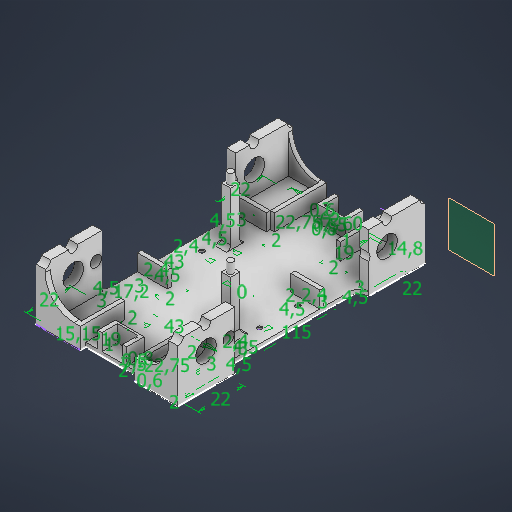
# Autodesk Inventor part: MainBody_thin
Saved by Autodesk Inventor 2026.1 (Build 301233000, 233)
## iProperties
Created: 2026-05-04
Part Number: MainBody_thin
Material: Generic
Document SubType Name: Modeling
Designer: 25adoh
Density: 1 g/cm^3
Appearance: Default
Author: 25adoh
Autodesk Inventor part; units mm, degrees
ref_plane "YZ Plane" through (0, 0, 0) normal (1, 0, 0) x (0, 1, 0)
ref_plane "XZ Plane" through (0, 0, 0) normal (0, 1, 0) x (-1, 0, 0)
ref_plane "XY Plane" through (0, 0, 0) normal (0, 0, 1) x (1, 0, 0)
sketch "Sketch1" plane through (0, 0, 0) normal (0, 1, 0) x (-1, 0, 0)
  line L0 (0, 0) -> (-60, 0)
  line L1 (-60, 0) -> (-60, -115)
  line L2 (-60, -115) -> (0, -115)
  line L3 (0, -115) -> (0, 0)
  line L4 (0, 0) -> (4.5, 0)
  line L5 (4.5, 0) -> (4.5, -22)
  line L6 (4.5, -22) -> (0, -22)
  line L7 (0, -22) -> (0, 0)
  line L8 (-60, 0) -> (-64.5, 0)
  line L9 (-64.5, 0) -> (-64.5, -22)
  line L10 (-64.5, -22) -> (-60, -22)
  line L11 (-60, -22) -> (-60, 0)
  line L12 (0, -115) -> (4.5, -115)
  line L13 (4.5, -115) -> (4.5, -93)
  line L14 (4.5, -93) -> (0, -93)
  line L15 (0, -93) -> (0, -115)
  line L16 (-60, -115) -> (-64.5, -115)
  line L17 (-64.5, -115) -> (-64.5, -93)
  line L18 (-64.5, -93) -> (-60, -93)
  line L19 (-60, -93) -> (-60, -115)
  line L20 (-44.8503, -96.0032) -> (-42.8503, -96.0032)
  line L21 (-42.8503, -96.0032) -> (-42.8503, -115)
  line L22 (-15.15, 0) -> (-15.15, -19)
  line L23 (-15.15, -19) -> (-17.15, -19)
  line L24 (-17.15, -19) -> (-17.15, 0)
  line L25 (-17.15, 0) -> (-15.15, 0)
  line L26 (-16.5, -115) -> (-14.5, -115)
  line L27 (-45.2, -115) -> (-42.8503, -115)
  line L28 (-46, -72.8) -> (-60, -72.8)
  line L29 (-46, -72.8) -> (-46, -70.8)
  line L30 (-46, -70.8) -> (-60, -70.8)
  line L31 (0, 0) -> (-15.15, 0)
  line L32 (-14.5, -42.2) -> (0, -42.2)
  line L33 (-43.5, 0) -> (-43.5, -22.75)
  line L34 (-45.5, 0) -> (-45.5, -22.75)
  line L35 (-45.5, -22.75) -> (-43.5, -22.75)
  line L36 (-43.5, -22.75) -> (-43.5, -24.75)
  line L37 (-43.5, 0) -> (-45.5, 0)
  line L38 (-43.5, -24.75) -> (-60, -24.75)
  line L39 (-45.5, -22.75) -> (-60, -22.75)
  line L40 (-14.5, -115) -> (-14.5, -92.25)
  line L41 (-14.5, -92.25) -> (0, -92.25)
  line L42 (-16.5, -115) -> (-16.5, -92.25)
  line L43 (-16.5, -92.25) -> (-14.5, -92.25)
  line L44 (-16.5, -92.25) -> (-16.5, -90.25)
  line L45 (-16.5, -90.25) -> (0, -90.25)
  line L46 (-45.5, 0) -> (-45.5, 0.6)
  line L47 (-60, 0) -> (-60, 0.6)
  line L48 (-60, 0.6) -> (-45.5, 0.6)
  line L49 (-60, 0.6) -> (-60, 2.6)
  line L50 (-60, 2.6) -> (-43.5, 2.6)
  line L51 (-43.5, 2.6) -> (-43.5, 0)
  line L52 (-16.5, -115) -> (-16.5, -115.6)
  line L53 (-16.5, -115.6) -> (0, -115.6)
  line L54 (-16.5, -115.6) -> (-16.5, -117.6)
  line L55 (-16.5, -117.6) -> (0, -117.6)
  line L56 (0, -117.6) -> (0, -115.6)
  line L57 (0, -115.6) -> (0, -115)
  line L58 (-14.5, -115) -> (-14.5, -115.6)
  line L59 (-17.15, 0) -> (0, 0)
  line L60 (0, 0) -> (0, 2.6)
  line L61 (0, 2.6) -> (-17.15, 2.6)
  line L62 (-17.15, 2.6) -> (-17.15, 0)
  line L63 (-42.8503, -115) -> (-60, -115)
  line L64 (-60, -115) -> (-60, -117.6)
  line L65 (-60, -117.6) -> (-42.8503, -117.6)
  line L66 (-42.8503, -117.6) -> (-42.8503, -115)
  line L67 (-44.8503, -96.0032) -> (-44.8503, -115)
  line L68 (-14.5, -42.2) -> (-14.5, -44.2)
  line L69 (-14.5, -44.2) -> (0, -44.2)
  line L70 (-35, -115) -> (-35, 0)
  line L71 (-64.5, -22) -> (-60, -22)
  line L72 (-60, -22) -> (-60, -25)
  line L73 (-60, -25) -> (-64.5, -25)
  line L74 (-64.5, -25) -> (-64.5, -22)
  line L75 (-64.5, -93) -> (-60, -93)
  line L76 (-60, -93) -> (-60, -90)
  line L77 (-60, -90) -> (-64.5, -90)
  line L78 (-64.5, -90) -> (-64.5, -93)
  line L79 (4.5, -22) -> (0, -22)
  line L80 (0, -22) -> (0, -25)
  line L81 (0, -25) -> (4.5, -25)
  line L82 (4.5, -25) -> (4.5, -22)
  line L83 (4.5, -93) -> (0, -93)
  line L84 (0, -93) -> (0, -90)
  line L85 (0, -90) -> (4.5, -90)
  line L86 (4.5, -90) -> (4.5, -93)
  line L87 (-64.5, 0) -> (-60, 0)
  line L88 (-60, 0) -> (-60, 2.6)
  line L89 (-60, 2.6) -> (-64.5, 2.6)
  line L90 (-64.5, 2.6) -> (-64.5, 0)
  line L91 (0, 2.6) -> (4.5, 2.6)
  line L92 (4.5, 2.6) -> (4.5, 0)
  line L93 (4.5, 0) -> (0, 0)
  line L94 (0, 0) -> (0, 2.6)
  line L95 (0, -117.6) -> (4.5, -117.6)
  line L96 (4.5, -117.6) -> (4.5, -115)
  line L97 (4.5, -115) -> (0, -115)
  line L98 (0, -115) -> (0, -117.6)
  line L99 (-64.5, -115) -> (-60, -115)
  line L100 (-60, -115) -> (-60, -117.6)
  line L101 (-60, -117.6) -> (-64.5, -117.6)
  line L102 (-64.5, -117.6) -> (-64.5, -115)
  line L103 (-25, 0) -> (-35, 0)
  line L104 (-35, 0) -> (-35, -7.5)
  line L105 (-35, -7.5) -> (-25, -7.5)
  line L106 (-25, -7.5) -> (-25, 0)
  line L107 (-35, -7.5) -> (-35, -6.7)
  line L108 (-35, -5.7) -> (-35, -6.7)
  line L109 (-25, 0) -> (-23, 0)
  line L110 (-35, -7.5) -> (-37, -7.5)
  line L111 (-37, -7.5) -> (-37, 0)
  line L112 (-37, 0) -> (-35, 0)
  line L113 (-35, 0) -> (-35, -7.5)
  line L114 (-35, -6.7) -> (-35.3, -6.7)
  line L115 (-35, -6.5) -> (-35, -6.7)
  line L116 (-37, -7.5) -> (-23, -7.5)
  line L117 (-23, -8.5) -> (-37, -8.5)
  line L118 (-37, -8.5) -> (-37, -7.5)
  line L119 (-35, -6.7) -> (-35.5, -6.7)
  line L120 (-35.5, -6.7) -> (-35.5, -5.7)
  line L121 (-35.5, -5.7) -> (-35, -5.7)
  line L122 (-35, -5.7) -> (-35, -6.7)
  line L123 (-15.15, 0) -> (0, 0)
  line L124 (0, -25) -> (0, -42.2)
  line L125 (-23, -8.5) -> (-23, 0)
  line L126 (-25, -115) -> (-25, 0)
  circle A0 centre (-7, -66.5) radius 1.2
  circle A1 centre (-7, -48.5) radius 1.2
  circle A2 centre (-53.3, -48.2) radius 1.2
  circle A3 centre (-53.3, -66.8) radius 1.2
  line L127 (-51.5, -79) -> (-8.5, -79)
  line L128 (-8.5, -79) -> (-8.5, -36)
  line L129 (-8.5, -36) -> (-51.5, -36)
  line L130 (-51.5, -36) -> (-51.5, -79)
  line L131 (-51.5, -79) -> (-8.5, -36) construction
  line L132 (-8.5, -79) -> (-51.5, -36) construction
  circle A4 centre (-11.25, -38.75) radius 1.5
  circle A5 centre (-11.25, -38.75) radius 2.25
  line L133 (-9, -41) -> (-13.5, -41)
  line L134 (-13.5, -41) -> (-13.5, -36.5)
  line L135 (-13.5, -36.5) -> (-9, -36.5)
  line L136 (-9, -36.5) -> (-9, -41)
  circle A6 centre (-48.75, -38.75) radius 1.5
  circle A7 centre (-48.75, -38.75) radius 2.25
  line L137 (-51, -41) -> (-46.5, -41)
  line L138 (-46.5, -41) -> (-46.5, -36.5)
  line L139 (-46.5, -36.5) -> (-51, -36.5)
  line L140 (-51, -36.5) -> (-51, -41)
  circle A8 centre (-48.75, -76.25) radius 1.5
  circle A9 centre (-48.75, -76.25) radius 2.25
  line L141 (-46.5, -74) -> (-51, -74)
  line L142 (-51, -74) -> (-51, -78.5)
  line L143 (-51, -78.5) -> (-46.5, -78.5)
  line L144 (-46.5, -78.5) -> (-46.5, -74)
  circle A10 centre (-11.25, -76.25) radius 1.5
  circle A11 centre (-11.25, -76.25) radius 2.25
  line L145 (-13.5, -74) -> (-9, -74)
  line L146 (-9, -74) -> (-9, -78.5)
  line L147 (-9, -78.5) -> (-13.5, -78.5)
  line L148 (-13.5, -78.5) -> (-13.5, -74)
  line L149 (-14.5, -92.25) -> (-14.5, -90.25)
  line L150 (-45.5, -22.75) -> (-45.5, -24.75)
  line L151 (-46.5, -67.8) -> (-51, -67.8)
  line L152 (-51, -67.8) -> (-51, -63.3)
  line L153 (-51, -63.3) -> (-46.5, -63.3)
  line L154 (-46.5, -63.3) -> (-46.5, -67.8)
  line L155 (-13.5, -47.2) -> (-9, -47.2)
  line L156 (-9, -47.2) -> (-9, -51.7)
  line L157 (-9, -51.7) -> (-13.5, -51.7)
  line L158 (-13.5, -51.7) -> (-13.5, -47.2)
  line L159 (-25, -115) -> (-25, -107.5)
  line L160 (-25, -107.5) -> (-35, -107.5)
  line L161 (-35, -107.5) -> (-35, -115)
  line L162 (-25, -107.5) -> (-25, -108.3)
  line L163 (-25, -109.3) -> (-25, -108.3)
  line L164 (-35, -115) -> (-37, -115)
  line L165 (-25, -107.5) -> (-23, -107.5)
  line L166 (-23, -107.5) -> (-23, -115)
  line L167 (-23, -115) -> (-25, -115)
  line L168 (-25, -115) -> (-25, -107.5)
  line L169 (-25, -108.3) -> (-24.7, -108.3)
  line L170 (-25, -108.5) -> (-25, -108.3)
  line L171 (-23, -107.5) -> (-37, -107.5)
  line L172 (-37, -106.5) -> (-23, -106.5)
  line L173 (-23, -106.5) -> (-23, -107.5)
  line L174 (-25, -108.3) -> (-24.5, -108.3)
  line L175 (-24.5, -108.3) -> (-24.5, -109.3)
  line L176 (-24.5, -109.3) -> (-25, -109.3)
  line L177 (-25, -109.3) -> (-25, -108.3)
  line L178 (-37, -106.5) -> (-37, -115)
  line L179 (-30, -57.5) -> (-30, -57.5)
  point P0 (-60, -93)
  point P1 (0, -93)
  point P2 (0, -24.2)
  point P3 (-35, -130)
  point P4 (-44.8503, -115)
  point P5 (-30, -67.5)
  point P6 (-30, -57.5)
  point P7 (-30, -57.5)
  point P8 (-12.75, -40.25)
  point P9 (-35, -8.5)
  point P10 (-25, -115)
  point P11 (-37, -115)
  point P12 (-35, -107.5)
  point P13 (-25, -107.5)
  point P14 (-25, -108.3)
  point P15 (-25, -109.3)
  point P16 (-23, -115)
  point P17 (-25, -115)
  point P18 (-25, -106.5)
  point P19 (-25, -107.5)
  point P20 (-35, -106.5)
  point P21 (-35, -115)
  dimension "d0" = 60
  dimension "d1" = 115
  dimension "d2" = 4.5
  dimension "d3" = 22
  dimension "d4" = 4.5
  dimension "d5" = 22
  dimension "d6" = 4.5
  dimension "d7" = 22
  dimension "d8" = 4.5
  dimension "d9" = 22
  dimension "d64" = 14.8
  dimension "d66" = 19
  dimension "d67" = 2
  dimension "d74" = 19
  dimension "d75" = 2
  dimension "d100" = 2
  dimension "d107" = 22.75
  dimension "d108" = 2
  dimension "d109" = 22.75
  dimension "d110" = 2
  dimension "d111" = 0.6
  dimension "d112" = 2
  dimension "d113" = 0.6
  dimension "d114" = 2
  dimension "d148" = 2
  dimension "d165" = 3
  dimension "d166" = 3
  dimension "d167" = 3
  dimension "d168" = 3
  dimension "d175" = 7.5
  dimension "d176" = 0.8
  dimension "d180" = 2
  dimension "d182" = 1
  dimension "d183" = 0.5
  dimension "d186" = 15.15
  dimension "d190" = 17.2
  dimension "d196" = 2.4
  dimension "d197" = 2.4
  dimension "d198" = 2.4
  dimension "d199" = 43
  dimension "d200" = 43
  dimension "d201" = 3
  dimension "d202" = 3
  dimension "d203" = 4.5
  dimension "d204" = 3
  dimension "d205" = 4.5
  dimension "d206" = 4.5
  dimension "d207" = 4.5
  dimension "d209" = 2.4
  dimension "d215" = 7.5
  dimension "d216" = 0.8
  dimension "d217" = 2
  dimension "d218" = 1
  dimension "d219" = 0.5
  dimension "d220" = 0
  constraints: 356 end point, 58 parallel, 44 perpendicular, 37 horizontal, 20 point on line, 18 vertical, 12 centre point, 4 coincident, 2 collinear, 2 midpoint, 20 other
  measures "d0" distance of L2.end L1.end
  measures "d1" distance of L1.end L1.start
  measures "d2" distance of L5.end L6.end
  measures "d3" distance of L4.end L5.end
  measures "d4" distance of L10.end L9.end
  measures "d5" distance of L9.end L8.end
  measures "d6" distance of L14.end L13.end
  measures "d7" distance of L13.end L12.end
  measures "d8" distance of L17.end L18.end
  measures "d9" distance of L16.end L17.end
  measures "d64" distance of L1.end L27.start
  measures "d66" distance of L27.start L20.start
  measures "d67" distance of L20.start L20.end
  measures "d74" distance of L22.start L22.end
  measures "d75" distance of L22.end L23.end
  measures "d100" distance of L28.start L29.end
  measures "d107" distance of L33.start L33.end
  measures "d108" distance of L33.end L36.end
  measures "d109" distance of L26.end L40.end
  measures "d110" distance of L42.end L44.end
  measures "d111" distance of L34.start L46.end
  measures "d112" distance of L47.end L49.end
  measures "d113" distance of L26.start L52.end
  measures "d114" distance of L52.end L54.end
  measures "d148" distance of L32.start L68.end
  measures "d165" distance of L71.end L72.end
  measures "d166" distance of L76.end L75.end
  measures "d167" distance of L80.end L79.end
  measures "d168" distance of L83.end L84.end
  measures "d175" distance of L104.end L103.end
  measures "d176" distance of L104.end L107.end
  measures "d180" distance of L111.end L112.end
  measures "d182" distance of L116.end L117.start
  measures "d183" distance of L120.end L121.end
  measures "d186" distance of L4.start L22.start
  measures "d190" distance of L80.end L32.end
  measures "d196" diameter of A0
  measures "d197" diameter of A2
  measures "d198" diameter of A3
  measures "d199" distance of L129.end L128.end
  measures "d200" distance of L128.end L127.end
  measures "d201" diameter of A4
  measures "d202" diameter of A6
  measures "d203" diameter of A7
  measures "d204" diameter of A8
  measures "d205" diameter of A11
  measures "d206" distance of L151.end L152.end
  measures "d207" distance of L155.end L156.end
  measures "d209" diameter of A1
  measures "d215" distance of L160.start L159.start
  measures "d216" distance of L160.start L177.end
  measures "d217" distance of L167.start L168.start
  measures "d218" distance of L171.end L178.start
  measures "d219" distance of L175.end L177.start
  measures "d220" distance of L179.start L179.end
extrude "Extrusion1" add sketch "Sketch1" along normal blind 2 contours L3 L32 L128 L129 L126 L117 L125 L0 L24 L23 L22 | L22 L23 L24 L0 | L125 L116 L106 L0 | L3 L69 L128 L32 | L106 L105 L70 L0 | L125 L117 L126 L116 | L3 L45 L44 L42 L2 L166 L173 L172 L126 L127 L128 L69 | L128 L69 L68 L32 | L32 L68 L69 L128 L127 L126 L129 | L70 L121 L120 L119 L114 L110 L111 L0 | L126 L117 L70 L105 | L111 L118 L117 L70 L129 L130 L30 L1 L38 L36 L33 L0 | L70 L114 L119 L120 L121 | L70 L117 L118 L110 | L126 L129 L70 L117 | L3 L41 L149 L45 | L126 L127 L70 L129 | L33 L35 L34 L0 | L0 L46 L48 L49 L50 L51 | L3 L2 L40 L41 | L149 L43 L44 L45 | L126 L172 L70 L127 | L70 L127 L130 L28 L29 L30 L129 | L34 L39 L1 L0 | L0 L47 L48 L46 | L36 L38 L150 L35 | L40 L2 L42 L43 | L172 L173 L165 L126 | L126 L160 L70 L172 | L70 L172 L178 L2 L21 L20 L67 L1 L28 L130 L127 | L150 L38 L1 L39 | L57 L53 L58 L2 | L58 L53 L52 L2 | L165 L166 L2 L126 L176 L175 L174 L169 | L126 L2 L70 L160 | L70 L171 L178 L172 | L130 L28 L1 L30 | L30 L29 L28 L130 | L56 L55 L54 L53 | L169 L174 L175 L176 L126 | L70 L2 L178 L171 | L2 L67 L20 L21 | A0 | A1 | A2 | A3 | A4 | A5 | L136 L133 A5 | A5 L135 L136 | A5 L134 L135 | L133 L134 A5 | A6 | A7 | L138 L137 A7 | A7 L139 L138 | A7 L140 L139 | L137 L140 A7 | A8 | A9 | L144 L143 A9 | A9 L141 L144 | A9 L142 L141 | L143 L142 A9 | A10 | A11 | L146 L147 A11 | A11 L145 L146 | A11 L148 L145 | L147 L148 A11 | L151 L152 L153 L154 | L155 L156 L157 L158
extrude "Extrusion2" add sketch "Sketch1" along normal blind 28 contours L4 L5 L6 L3 | L6 L82 L81 L3 | L85 L86 L14 L3 | L13 L12 L3 L14 | L1 L10 L9 L8 | L1 L73 L74 L10 | L1 L18 L78 L77 | L1 L16 L17 L18
sketch "Sketch2" plane through (64.5, 0, 0) normal (1, 0, 0) x (0, 0, -1)
  line L0 (0, 28) -> (25, 28) projected
  line L1 (22, 0) -> (22, 28) projected
  line L2 (0, 28) -> (0, 5)
  line L3 (0, 5) -> (22, 5)
  line L4 (0, 28) -> (22, 5)
  line L5 (22, 0) -> (22, 28) projected
  line L6 (0, 5) -> (22, 28)
  circle A0 centre (11, 16.5) radius 5
  line L7 (88, 28) -> (110, 28)
  line L8 (88, 0) -> (88, 28)
  line L9 (110, 0) -> (110, 28)
  line L10 (88, 28) -> (88, 5)
  line L11 (88, 5) -> (110, 5)
  line L12 (88, 28) -> (110, 5)
  line L13 (110, 0) -> (110, 28)
  line L14 (88, 5) -> (110, 28)
  circle A1 centre (99, 16.5) radius 5
  line L15 (115, 0) -> (115, 28) projected
  line L16 (0, 28) -> (0, 5)
  line L17 (12.5, 28) -> (11.25, 28) construction
  circle A2 centre (11, 27.75) radius 2.25
  circle A3 centre (99, 27.75) radius 2.25
  circle A4 centre (22, 16.5) radius 2.75
  circle A5 centre (88, 16.5) radius 2.75
  point P0 (118, 16.5)
  dimension "d14" = 23
  dimension "d15" = 10
  dimension "d16" = 23
  dimension "d17" = 10
  dimension "d60" = 4.5
  dimension "d61" = 4.5
  dimension "d115" = 5.5
  dimension "d214" = 5.5
  constraints: 28 end point, 6 centre point, 4 midpoint, 4 point on line, 3 perpendicular, 1 coincident, 1 horizontal
  measures "d14" distance of L0.start L2.end
  measures "d15" diameter of A0
  measures "d16" distance of L7.start L10.end
  measures "d17" diameter of A1
  measures "d60" diameter of A2
  measures "d61" diameter of A3
  measures "d115" diameter of A4
  measures "d214" diameter of A5
extrude "Extrusion3" cut sketch "Sketch2" against normal up to surface (69 mm away) contours A2 L0 | L0 A2 | A0 L6 L4 | L4 L6 A0 | L6 L4 A0 | L6 A0 L4 | A4 L1 | L1 A4 | A3 L7 | L7 A3 | A5 L8 | L8 A5 | A1 L14 L12 | L12 L14 A1 | L14 A1 L12 | L12 A1 L14
ref_plane "Work Plane1" through (64.5, 0, -140) normal (0, 0, -1) x (-1, 0, 0)
sketch "Sketch5" plane through (64.5, 0, -140) normal (0, 0, -1) x (-1, 0, 0)
  line L0 (42, 5) -> (42, 20) projected
  line L1 (4.5, 2) -> (4.5, 28) projected
  line L2 (0, 28) -> (4.5, 28) projected
  line L3 (0, 0) -> (0, 28) projected
  line L4 (34.5, 20) -> (34.5, 5)
  line L5 (27, 5) -> (42, 5) projected
  line L6 (34.5, 5) -> (34.5, 13)
  line L7 (30.5, 13) -> (38.5, 13)
  line L8 (38.5, 13) -> (38.5, 5)
  line L9 (30.5, 13) -> (30.5, 5)
  line L10 (0, 0) -> (48, 0) projected
  line L11 (48, 0) -> (48, 2) projected
  line L12 (4.5, 2) -> (48, 2) projected
  point P0 (64.5, 0)
  point P1 (42, 5)
  dimension "d40" = 8
  dimension "d41" = 8
  constraints: 10 end point, 3 point on line, 2 midpoint, 2 perpendicular, 1 horizontal
  measures "d40" distance of L4.end L6.end
  measures "d41" distance of L7.start L7.end
extrude "Extrusion6" cut sketch "Sketch5" against normal blind 6 contours L7 L8 L5 L4 | L4 L5 L9 L7
extrude "Extrusion7" add sketch "Sketch1" along normal blind 10 contours L60 L91 L92 L4 | L0 L62 L61 L60 | L22 L23 L24 L0 | L3 L69 L128 L32 | L128 L69 L68 L32 | L3 L41 L149 L45 | L33 L35 L34 L0 | L0 L46 L48 L49 L50 L51 | L40 L2 L42 L43 | L96 L95 L56 L57 L12 | L8 L90 L89 L49 L47 | L150 L38 L1 L39 | L58 L53 L52 L2 | L130 L28 L1 L30 | L30 L29 L28 L130 | L56 L55 L54 L53 | L66 L65 L64 L2 | L2 L67 L20 L21 | L64 L101 L102 L16
extrude "Extrusion8" add sketch "Sketch1" along normal blind 28 contours A6 | A7 | L138 L137 A7 | A7 L139 L138 | A7 L140 L139 | L137 L140 A7 | A10 | A11 | L146 L147 A11 | A11 L145 L146 | A11 L148 L145 | L147 L148 A11
extrude "Extrusion9" add sketch "Sketch1" along normal blind 33 contours A6 | A10
fillet "Fillet3" radius 4.5 4 edges at (0, 1, -25) (0, 1, -90) (60, 1, -90) (60, 1, -25)
extrude "Extrusion12" add sketch "Sketch1" along normal blind 5.5 contours L3 L2 L40 L41 | L34 L39 L1 L0 | L0 L47 L48 L46 | L57 L53 L58 L2 | L56 L55 L54 L53
extrude "Extrusion14" cut sketch "Sketch1" along normal up to surface (2 mm away) contours A0 | A1 | A2 | A3
fillet "Fillet4" radius 1.5 4 edges at (54.5, 0, -48.2) (54.5, 0, -66.8) (8.2, 0, -48.5) (8.2, 0, -66.5)
fillet "Fillet5" radius 2 6 edges at (11.25, 2, -74) (9, 2, -76.25) (11.25, 2, -78.5) (48.75, 2, -41) (48.75, 2, -36.5) (51, 2, -38.75)
extrude "Extrusion15" add sketch "Sketch1" along normal blind 25.4 contours L60 L91 L92 L4 | L96 L95 L56 L57 L12 | L8 L90 L89 L49 L47 | L64 L101 L102 L16
fillet "Fillet6" radius 2.6 4 edges at (-2.25, 25.4, 0) (62.25, 25.4, 0) (-2.25, 25.4, -115) (62.25, 25.4, -115)
fillet "Fillet7" radius 14 4 edges at (60, 10, 1.6) (0, 10, 1.3) (0, 10, -116.6) (60, 10, -116.3)
extrude "Extrusion16" add sketch "Sketch1" along normal blind 10 contours L125 L116 L106 L0 | L125 L117 L126 L116 | L70 L121 L120 L119 L114 L110 L111 L0 | L126 L117 L70 L105 | L70 L117 L118 L110 | L172 L173 L165 L126 | L126 L160 L70 L172 | L165 L166 L2 L126 L176 L175 L174 L169 | L70 L171 L178 L172 | L70 L2 L178 L171
body "Solid1"
